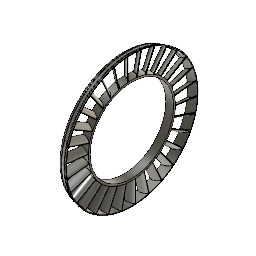
petrol_turbine_four_eng_model (Autodesk Fusion 360 design; units mm, degrees)
Autodesk Fusion 360 part; units mm, degrees
sketch "Sketch1" plane through (0, 0, 0) normal (1, 0, 0) x (0, 1, 0)
  circle A0 centre (0, 0) radius 104.57
  circle A1 centre (0, 0) radius 109.57
  dimension "d1" = 209.14
  dimension "d2" = 5
  constraint coincident A0.centre A1.centre
  constraint concentric A0 A1
  measures "d1" diameter of A0
  measures "d2" distance of A0 A1
extrude "Extrude1" add sketch "Sketch1" along normal blind 20 makes body 1
sketch "Sketch2" plane through (0, 0, 0) normal (0, 1, 0) x (1, 0, 0)
  line L0 (20, -109.57) -> (20, 109.57)
  line L1 (0, -109.57) -> (0, 109.57)
  line L2 (0, 0) -> (0, -231.8481) construction
  line L3 (20, 0) -> (20, -234.6005) construction
  line L4 (0, -159.21) -> (20, -164.57)
  line L5 (20, -166.64) -> (20, -164.57)
  line L6 (0, -161.28) -> (0, -159.21)
  arc A0 (4.0341, -162.3611) -> (5.9659, -162.8789) centre (5, -162.62) ccw
  line L7 (0, -161.28) -> (4.0341, -162.3611)
  arc A1 (14.0341, -165.0411) -> (15.9659, -165.5589) centre (15, -165.3) ccw
  line L8 (5.9659, -162.8789) -> (14.0341, -165.0411)
  line L9 (15.9659, -165.5589) -> (20, -166.64)
  dimension "d5" = 164.57
  dimension "d6" = 159.21
  dimension "d7" = 166.64
  dimension "d8" = 161.28
  dimension "d9" = 2
  dimension "d10" = 2
  dimension "d11" = 5
  dimension "d12" = 5
  constraint coincident L2.start origin
  constraint parallel L0 L2
  constraint midpoint L0 L3.start
  constraint parallel L0 L3
  constraint coincident L2 L4.start
  constraint coincident L3 L4.end
  constraint coincident L2 L6.start
  constraint coincident L3 L5.start
  constraint coincident A0.centre L7
  constraint coincident A1.centre L7
  constraint coincident A0.end L7
  constraint collinear L7 L8
  constraint coincident A1.end L8
  constraint collinear L8 L9
  measures "d5" distance of L3.start L4.end
  measures "d6" distance of L2.start L4.start
  measures "d7" distance of L3.start L5.start
  measures "d8" distance of L2.start L6.start
  measures "d9" diameter of A0
  measures "d10" diameter of A1
  measures "d11" distance of L3 A1.centre
  measures "d12" distance of L2 A0.centre
revolve "Revolve1" add sketch "Sketch2" angle 360 about axis through (1.75, 0, 0) along (1, 0, 0) separate body makes body 2
sketch "Sketch3" plane through (0, 0, 0) normal (0, 1, 0) x (1, 0, 0)
  line L0 (0, 161.28) -> (0, -161.28)
  line L1 (20, 166.64) -> (20, -166.64)
  line L2 (15.9659, -165.5589) -> (20, -166.64)
  line L3 (15.9659, 165.5589) -> (20, 166.64)
  arc A0 (14, -165.3) -> (15.9659, -165.5589) centre (15, -165.3) ccw
  arc A1 (15.9659, 165.5589) -> (14, 165.3) centre (15, 165.3) ccw
  line L4 (14, 165.3) -> (14, 165.032)
  line L5 (14, -165.032) -> (14, -165.3)
  line L6 (5.9659, -162.8789) -> (14, -165.032)
  line L7 (5.9659, 162.8789) -> (14, 165.032)
  arc A2 (4, -162.62) -> (5.9659, -162.8789) centre (5, -162.62) ccw
  arc A3 (5.9659, 162.8789) -> (4, 162.62) centre (5, 162.62) ccw
  line L8 (4, 162.62) -> (4, 162.352)
  line L9 (4, -162.352) -> (4, -162.62)
  line L10 (0, -161.28) -> (4, -162.352)
  line L11 (0, 161.28) -> (4, 162.352)
  line L12 (0, 161.28) -> (0, 174.5237)
  line L13 (0, 161.28) -> (4, 162.352)
  line L14 (5.9659, 162.8789) -> (14, 165.032)
  line L15 (15.9659, 165.5589) -> (20, 166.64)
  line L16 (20, 166.64) -> (20, 174.5237)
  line L17 (20, 174.5237) -> (0, 174.5237)
  arc A4 (5.9659, 162.8789) -> (4, 162.62) centre (5, 162.62) ccw
  arc A5 (15.9659, 165.5589) -> (14, 165.3) centre (15, 165.3) ccw
  dimension "d14" = 2
  dimension "d15" = 2
  constraint coincident L0.start L11.start
  constraint parallel L0 L12
  constraint coincident L8.end L11.end
  constraint coincident L7.start A3.start
  constraint coincident L4.end L7.end
  constraint coincident L3.start A1.start
  constraint coincident L1.start L3.end
  constraint parallel L1 L16
  constraint perpendicular L1 L17
  constraint concentric A3 A4
  constraint concentric A1 A5
  measures "d14" diameter of A4
  measures "d15" diameter of A5
sketch "Sketch4" plane through (0, 0, 0) normal (0, 0, 1) x (1, 0, 0)
  line L0 (20, 166.64) -> (20, -166.64)
  arc A0 (19.8634, -9.4954) -> (0.9723, 0.9996) centre (1.5599, -20.1922) ccw
  arc A1 (18.1366, -10.5046) -> (1.0277, -0.9996) centre (1.5599, -20.1922) ccw
  line L1 (1.0277, -0.9996) -> (0.9723, 0.9996)
  line L2 (18.1366, -10.5046) -> (19.8634, -9.4954)
  point P0 (1, 0)
  point P1 (19, -10)
  point P2 (20, 0)
  dimension "d16" = 1
  dimension "d17" = 1
  dimension "d18" = 10
  measures "d16" distance of origin P0
  measures "d17" distance of P1 L0
  measures "d18" vertical distance of P1 P2
extrude "Extrude2" add sketch "Sketch4" along normal blind 167 separate body makes body 3
fillet "Fillet1" radius 1 4 edges at (19.8634, -9.4954, 83.5) (18.1366, -10.5046, 83.5) (1.0277, -0.9996, 83.5) (0.9723, 0.9996, 83.5) on bodies 3
pattern_circular "C-Pattern1" count 30 over 360 about axis through (1.75, 0, 0) along (1, 0, 0) of "Extrude2", "Fillet1" makes body 4 at (16.185, -27.8863, 107.8932) makes body 5 at (18.1658, -51.6904, 98.8555) makes body 6 at (18.1658, -71.114, 85.9482) makes body 7 at (14.7059, -85.1191, 71.8508) makes body 8 at (16.185, -98.8399, 51.471) makes body 9 at (18.1658, -108.0515, 27.7338) makes body 10 at (16.185, -111.2298, 6.8193) makes body 11 at (16.185, -110.217, -16.4557) makes body 12 at (16.185, -104.3872, -39.0115) makes body 13 at (18.1658, -92.9108, -61.7404) makes body 14 at (5.9103, -83.1092, -74.0829) makes body 15 at (18.1658, -59.7662, -94.1929) makes body 16 at (8.7363, -45.0606, -101.8072) makes body 17 at (18.1658, -16.2874, -110.3586) makes body 18 at (3.9765, -0.8696, -111.3333) makes body 19 at (3.9765, 22.2969, -109.0812) makes body 20 at (14.7059, 48.5358, -100.26) makes body 21 at (18.1658, 71.114, -85.9482) makes body 22 at (5.9103, 82.3644, -74.9102) makes body 23 at (14.7059, 98.1976, -52.5834) makes body 24 at (16.185, 107.3814, -29.7963) makes body 25 at (16.185, 111.2298, -6.8193) makes body 26 at (16.185, 110.217, 16.4557) makes body 27 at (18.1658, 103.717, 41.074) makes body 28 at (16.185, 93.9951, 59.8623) makes body 29 at (3.0009, 42.0099, 36.5358) makes body 30 at (18.1658, 59.7662, 94.1929) makes body 31 at (18.1658, 38.8763, 104.5607) makes body 32 at (3.9765, 23.9981, 108.7196)
revolve "Revolve2" cut sketch "Sketch3" angle 360 about axis through (1.75, 0, 0) along (1, 0, 0) contours L3 A1 L4 L7 A3 L8 L11 L12 L13 L14 L15 L16 L17 A4 A5 bodies 3 4 5 6 7 8 9 10 11 12 13 14 15 16 17 18 19 20 21 22 23 24 25 26 27 28 29 30 31 32
sketch "Sketch5" plane through (20, 0, 0) normal (1, 0, 0) x (0, 1, 0)
  circle A0 centre (0, 0) radius 104.57
  circle A1 centre (0, 0) radius 109.57
  circle A2 centre (0, 0) radius 104.57
  dimension "d29" = 209.14
  constraint coincident A0.centre A1.centre
  measures "d29" diameter of A2
extrude "Extrude3" cut sketch "Sketch5" against normal blind 25 contours A0 A2 bodies 3 4 5 6 7 8 9 10 11 12 13 14 15 16 17 18 19 20 21 22 23 24 25 26 27 28 29 30 31 32
combine "Combine1" operation add target body 10 tool bodies 11 2 1 12 13 22 25 7 20 15 18 29 5 19 16 17 32 31 3 27 8 9 26 24 23 6 4 30 28 21 14
equation "d1 = ( 104.57 * 2 ) * 1 mm"
equation "d29 = ( 104.57 * 2 ) * 1 mm"
